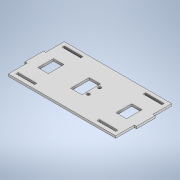
# Autodesk Inventor part: Level4 (Sensor + Schakelaar)
Saved by Autodesk Inventor 2020 (Build 240168000, 168)
## iProperties
Created: 2020-01-30
Part Number: Level4 (Sensor + Schakelaar)
Material: Generic
Document SubType Name: Modeling
Designer: jelte
Density: 1 g/cm^3
Appearance: Default
Mass: 29.3096 g
Surface Area: 219.611 cm^2
Volume: 29.3096 cm^3
Author: jelte
Autodesk Inventor part; units mm, degrees
ref_plane "YZ Plane" through (0, 0, 0) normal (1, 0, 0) x (0, 1, 0)
ref_plane "XZ Plane" through (0, 0, 0) normal (0, 1, 0) x (-1, 0, 0)
ref_plane "XY Plane" through (0, 0, 0) normal (0, 0, 1) x (1, 0, 0)
sketch "Sketch1" plane through (0, 0, 0) normal (0, 1, 0) x (-1, 0, 0)
  line L0 (71.1097, -38.0648) -> (71.1097, -13.0648)
  line L1 (71.1097, -13.0648) -> (74.1097, -13.0648)
  line L2 (74.1097, -13.0648) -> (74.1097, 11.9352)
  line L3 (74.1097, 11.9352) -> (71.1097, 11.9352)
  line L4 (71.1097, 11.9352) -> (71.1097, 36.9352)
  line L5 (-72.8903, -38.0648) -> (-72.8903, -13.0648)
  line L6 (-72.8903, 36.9352) -> (-72.8903, 11.9352)
  line L7 (-72.8903, -13.0648) -> (-75.8903, -13.0648)
  line L8 (-75.8903, -13.0648) -> (-75.8903, 11.9352)
  line L9 (-75.8903, 11.9352) -> (-72.8903, 11.9352)
  line L10 (71.1097, -38.0648) -> (-72.8903, -38.0648)
  line L11 (71.1097, 36.9352) -> (-72.8903, 36.9352)
  point P0 (0, 0)
  constraints: 24 end point, 5 perpendicular, 3 horizontal, 2 vertical
extrude "Extrusion1" add sketch "Sketch1" along normal blind 3
sketch "Sketch2" plane through (0, 3, 0) normal (0, 1, 0) x (1, 0, 0)
  line L0 (-71.1097, -36.9352) -> (72.8903, -36.9352) projected
  line L1 (-66.1097, -31.9352) -> (-56.1097, -31.9352)
  line L2 (-56.1097, -31.9352) -> (-56.1097, -28.9352)
  line L3 (-56.1097, -28.9352) -> (-66.1097, -28.9352)
  line L4 (-66.1097, -28.9352) -> (-66.1097, -31.9352)
  line L5 (72.8903, 38.0648) -> (-71.1097, 38.0648) projected
  line L6 (-56.1097, 30.0648) -> (-66.1097, 30.0648)
  line L7 (-66.1097, 30.0648) -> (-66.1097, 33.0648)
  line L8 (-66.1097, 33.0648) -> (-56.1097, 33.0648)
  line L9 (-56.1097, 33.0648) -> (-56.1097, 30.0648)
  line L10 (67.8903, 33.0648) -> (57.8903, 33.0648)
  line L11 (57.8903, 33.0648) -> (57.8903, 30.0648)
  line L12 (57.8903, 30.0648) -> (67.8903, 30.0648)
  line L13 (67.8903, 30.0648) -> (67.8903, 33.0648)
  line L14 (67.8903, -31.9352) -> (57.8903, -31.9352)
  line L15 (57.8903, -31.9352) -> (57.8903, -28.9352)
  line L16 (57.8903, -28.9352) -> (67.8903, -28.9352)
  line L17 (67.8903, -28.9352) -> (67.8903, -31.9352)
  point P0 (0, 0)
  constraints: 32 end point, 8 parallel, 4 horizontal, 4 perpendicular, 1 point on line
extrude "Extrusion2" cut sketch "Sketch2" against normal blind 30
sketch "Sketch3" plane through (0, 3, 0) normal (0, 1, 0) x (1, 0, 0)
  line L0 (72.8903, 38.0648) -> (-71.1097, 38.0648) projected
  line L1 (-71.1097, -36.9352) -> (72.8903, -36.9352) projected
  line L2 (-74.1097, 13.0648) -> (-74.1097, -11.9352) projected
  line L3 (75.8903, -11.9352) -> (75.8903, 13.0648) projected
  circle A0 centre (6.2215, -7.0252) radius 2
  circle A1 centre (6.2215, 8.1548) radius 2
  line L4 (2.4888, 13.0648) -> (-12.5112, 13.0648)
  line L5 (-12.5112, 13.0648) -> (-12.5112, -11.9352)
  line L6 (-12.5112, -11.9352) -> (2.4888, -11.9352)
  line L7 (2.4888, -11.9352) -> (2.4888, 13.0648)
  line L8 (-58.6097, -9.9352) -> (-44.6097, -9.9352)
  line L9 (-44.6097, -9.9352) -> (-44.6097, 11.0648)
  line L10 (-44.6097, 11.0648) -> (-58.6097, 11.0648)
  line L11 (-58.6097, 11.0648) -> (-58.6097, -9.9352)
  line L12 (60.3903, 11.0648) -> (46.3903, 11.0648)
  line L13 (46.3903, 11.0648) -> (46.3903, -9.9352)
  line L14 (46.3903, -9.9352) -> (60.3903, -9.9352)
  line L15 (60.3903, -9.9352) -> (60.3903, 11.0648)
  line L16 (-71.1097, -36.9352) -> (72.8903, -36.9352) projected
  point P0 (0, 0)
  dimension "d56" = 14
  dimension "d57" = 21
  dimension "d59" = 25
  dimension "d60" = 15
  dimension "d61" = 4
  dimension "d62" = 4
  dimension "d63" = 14
  dimension "d64" = 21
  constraints: 24 end point, 6 parallel, 3 horizontal, 3 perpendicular, 2 centre point
  measures "d56" distance of L9.end L10.end
  measures "d57" distance of L8.end L9.end
  measures "d59" distance of L4.end L5.end
  measures "d60" distance of L4.start L4.end
  measures "d61" diameter of A1
  measures "d62" diameter of A0
  measures "d63" distance of L12.start L12.end
  measures "d64" distance of L12.end L13.end
extrude "Extrusion3" cut sketch "Sketch3" against normal blind 10
sketch "Sketch4" plane through (0, 3, 0) normal (0, 1, 0) x (1, 0, 0)
  line L0 (-56.1097, 33.0648) -> (-41.1097, 33.0648)
  line L1 (-41.1097, 33.0648) -> (-41.1097, 29.924)
  line L2 (-41.1097, 29.924) -> (-56.1097, 29.924)
  line L3 (-56.1097, 29.924) -> (-56.1097, 33.0648)
  line L4 (57.8903, 30.0648) -> (57.8903, 33.0648) projected
  line L5 (57.8903, 33.0648) -> (42.8903, 33.0648)
  line L6 (42.8903, 33.0648) -> (42.8903, 29.924)
  line L7 (42.8903, 29.924) -> (57.8903, 29.924)
  line L8 (57.8903, 29.924) -> (57.8903, 33.0648)
  line L9 (-56.1097, -31.9352) -> (-41.1097, -31.9352)
  line L10 (-41.1097, -31.9352) -> (-41.1097, -28.9352)
  line L11 (-41.1097, -28.9352) -> (-56.1097, -28.9352)
  line L12 (-56.1097, -28.9352) -> (-56.1097, -31.9352)
  line L13 (57.8903, -31.9352) -> (57.8903, -28.9352) projected
  line L14 (57.8903, -28.9352) -> (42.8903, -28.9352)
  line L15 (42.8903, -28.9352) -> (42.8903, -31.9352)
  line L16 (42.8903, -31.9352) -> (57.8903, -31.9352)
  line L17 (57.8903, -31.9352) -> (57.8903, -28.9352)
  point P0 (0, 0)
  dimension "d67" = 15
  dimension "d68" = 15
  constraints: 32 end point, 8 parallel, 4 horizontal, 4 perpendicular, 1 point on line
  measures "d67" distance of L0.start L0.end
  measures "d68" distance of L4.end L5.end
extrude "Extrusion4" cut sketch "Sketch4" against normal blind 10
sketch "Sketch5" plane through (-41.1097, 3, -29.924) normal (0, 0, -1) x (-1, 0, 0)
  line L0 (15, -3) -> (0, -3) projected
  line L1 (0, 0) -> (15, 0) projected
  line L2 (15, -3) -> (0, -3)
  line L3 (0, -3) -> (0, 0)
  line L4 (0, 0) -> (15, 0)
  line L5 (15, 0) -> (15, -3)
  point P0 (-41.1097, -3)
  constraints: 8 end point, 2 parallel, 1 horizontal, 1 perpendicular
extrude "Extrusion5" add sketch "Sketch5" along normal blind 0.14
sketch "Sketch6" plane through (57.8903, 3, -29.924) normal (0, 0, -1) x (-1, 0, 0)
  line L0 (0, 0) -> (15, 0)
  line L1 (15, 0) -> (15, -3)
  line L2 (15, -3) -> (0, -3)
  line L3 (0, -3) -> (0, 0)
  point P0 (57.8903, -3)
  constraints: 8 end point, 2 parallel, 1 horizontal, 1 perpendicular
extrude "Extrusion6" add sketch "Sketch6" along normal blind 0.14
body "Solid1"
